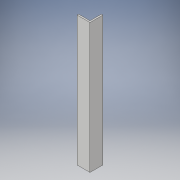
# Autodesk Inventor part: BumberGussetFront.ver1-1111-2020
Saved by Autodesk Inventor 2018 (Build 220112000, 112)
## iProperties
Created: 2020-01-29
Part Number: BumberGussetFront.ver1-1111-2020
Material: Generic
Document SubType Name: Modeling
Designer: JMHal
Density: 1 g/cm^3
Appearance: Default
Author: JMHal
Autodesk Inventor part; units mm, degrees
ref_plane "YZ Plane" through (0, 0, 0) normal (1, 0, 0) x (0, 1, 0)
ref_plane "XZ Plane" through (0, 0, 0) normal (0, 1, 0) x (-1, 0, 0)
ref_plane "XY Plane" through (0, 0, 0) normal (0, 0, 1) x (1, 0, 0)
sketch "Sketch1" plane through (0, 0, 0) normal (0, 1, 0) x (-1, 0, 0)
  line L0 (0, 0) -> (25.4, 0)
  line L1 (25.4, 0) -> (25.4, -25.4)
  line L2 (25.4, -25.4) -> (0, -25.4)
  line L3 (0, -25.4) -> (0, 0)
  line L4 (22.225, -3.175) -> (3.175, -3.175)
  line L5 (3.175, -3.175) -> (3.175, -22.225)
  line L6 (3.175, -22.225) -> (22.225, -22.225)
  line L7 (22.225, -22.225) -> (22.225, -3.175)
  line L8 (22.225, -3.175) -> (25.4, -3.175)
  line L9 (3.175, -22.225) -> (3.175, -25.4)
  dimension "d0" = 25.4
  dimension "d1" = 25.4
  dimension "d2" = 3.175
  constraints: 20 end point, 4 parallel, 3 perpendicular, 2 horizontal, 2 point on line, 3 other
  measures "d0" distance of L1.end L2.end
  measures "d1" distance of L0.end L1.end
  measures "d2" distance between parallel lines of L0 L4
extrude "Extrusion1" add sketch "Sketch1" along normal blind 254 contours L0 L1 L8 L4 L5 L9 L2 L3
body "Solid1"
